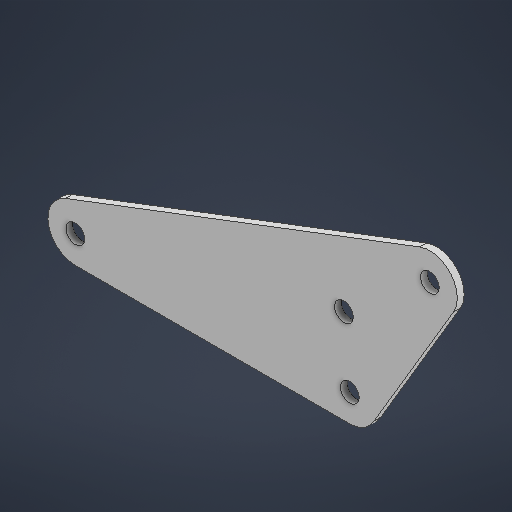
# Autodesk Inventor part: intakesupportpoly
Saved by Autodesk Inventor 2025.2 (Build 292293000, 293)
## iProperties
Created: 2025-03-29
Part Number: intakesupportpoly
Material: Generic
Document SubType Name: Modeling
Designer: roejo
Density: 1 g/cm^3
Appearance: Default
Author: roejo
Autodesk Inventor part; units mm, degrees
ref_plane "YZ Plane" through (0, 0, 0) normal (1, 0, 0) x (0, 1, 0)
ref_plane "XZ Plane" through (0, 0, 0) normal (0, 1, 0) x (-1, 0, 0)
ref_plane "XY Plane" through (0, 0, 0) normal (0, 0, 1) x (1, 0, 0)
sketch "Sketch1" plane through (0, 0, 0) normal (0, 0, 1) x (1, 0, 0)
  ellipse E0 centre (41.1667, 15.8884) end of major axis (43.1515, 16.8006) minor radius 2.1841
  ellipse E1 centre (21.2939, 0.0699) end of major axis (23.2787, 0.9821) minor radius 2.1841
  circle A0 centre (22.6398, -15.3868) radius 2.1844
  circle A1 centre (-40.8602, -15.3868) radius 2.1844
  circle A2 centre (-40.8602, -15.3868) radius 6.35
  circle A3 centre (22.6398, -15.3868) radius 6.35
  circle A4 centre (41.1667, 15.8884) radius 6.35
  line L0 (28.2205, -18.4164) -> (46.6296, 12.6513)
  line L1 (38.8163, 21.7874) -> (-43.1224, -9.4534)
  line L2 (-40.8602, -21.7368) -> (22.6398, -21.7368)
  point P0 (0, 0)
  dimension "d0" = 12.7
  dimension "d1" = 12.7
  dimension "d2" = 12.7
  constraints: 7 centre point, 6 end point, 6 point on circle, 3 coincident, 3 tangent
  measures "d0" diameter of A2
  measures "d1" diameter of A3
  measures "d2" diameter of A4
extrude "Extrusion1" add sketch "Sketch1" along normal blind 1.5875
body "Solid1"
